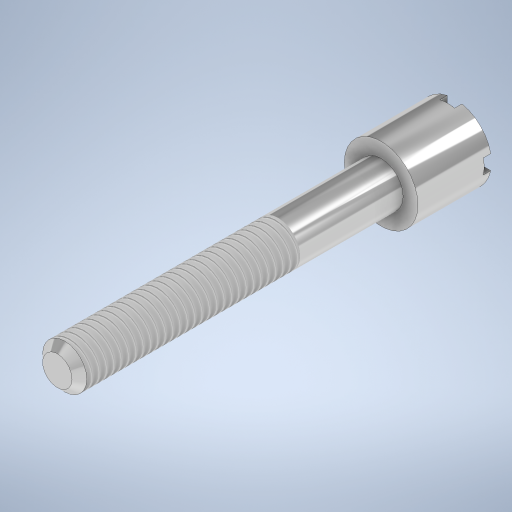
# Autodesk Inventor part: PARAFUSO
Saved by Autodesk Inventor 2023 (Build 270158000, 158)
## iProperties
Created: 2023-10-18
Part Number: PARAFUSO
Material: Genérico
Document SubType Name: Modeling
Designer: vinicius.sena
Density: 1 g/cm^3
Appearance: Padrão
Author: vinicius.sena
Autodesk Inventor part; units mm, degrees
ref_plane "YZ Plane" through (0, 0, 0) normal (1, 0, 0) x (0, 1, 0)
ref_plane "XZ Plane" through (0, 0, 0) normal (0, 1, 0) x (-1, 0, 0)
ref_plane "XY Plane" through (0, 0, 0) normal (0, 0, 1) x (1, 0, 0)
sketch "Esboço1" plane through (0, 0, 0) normal (0, 0, 1) x (1, 0, 0)
  circle A0 centre (0, 0) radius 2.5
  dimension "d0" = 5
  constraints: 1 centre point, 1 coincident
  measures "d0" diameter of A0
extrude "Extrusão1" add sketch "Esboço1" along normal blind 5
sketch "Esboço2" plane through (0, 0, 5) normal (0, 0, 1) x (1, 0, 0)
  circle A0 centre (0, 0) radius 1.5
  dimension "d3" = 3
  constraints: 1 centre point, 1 coincident
  measures "d3" diameter of A0
extrude "Extrusão2" add sketch "Esboço2" along normal blind 22
thread "Rosca1" size "M3x0.5" class "6g" standard "ANSI Metric M Profile" length 15 offset 7
sketch "Esboço3" plane through (0, 0, 0) normal (0, 0, -1) x (-1, 0, 0)
  point P0 (0, 0)
  point P1 (0, 0)
  dimension "d15" = 0
  dimension "d16" = 0
  measures "d15" distance of point (0, 0) point (0, 0)
  measures "d16" distance of point (0, 0) point (0, 0)
hole "Furo1" at (0, 0, 0) direction (0, 0, 1) diameter 2.459 depth 4 tip angle 118 thread size "M3x0.5" class "6H" standard "ANSI Metric M Profile"
sketch "Esboço4" plane through (0, 0, 0) normal (0, 0, -1) x (-1, 0, 0)
  line L0 (-0.5, -3) -> (0.5, -3)
  line L1 (0.5, -3) -> (0.5, 3)
  line L2 (0.5, 3) -> (-0.5, 3)
  line L3 (-0.5, 3) -> (-0.5, -3)
  line L4 (-0.5, -3) -> (0.5, 3) construction
  line L5 (0.5, -3) -> (-0.5, 3) construction
  line L6 (-3, -0.5) -> (3, -0.5)
  line L7 (3, -0.5) -> (3, 0.5)
  line L8 (3, 0.5) -> (-3, 0.5)
  line L9 (-3, 0.5) -> (-3, -0.5)
  line L10 (-3, -0.5) -> (3, 0.5) construction
  line L11 (3, -0.5) -> (-3, 0.5) construction
  point P0 (0, 0)
  point P1 (-0.5, -0.5)
  point P2 (-0.5, 0.5)
  point P3 (0.5, 0.5)
  point P4 (0.5, -0.5)
  dimension "d17" = 1
  dimension "d18" = 6
  dimension "d19" = 6
  dimension "d20" = 1
  constraints: 24 end point, 4 midpoint, 4 parallel, 2 horizontal, 2 perpendicular
  measures "d17" distance of L2.end L1.end
  measures "d18" distance of L1.end L0.end
  measures "d19" distance of L8.end L7.end
  measures "d20" distance of L7.end L6.end
extrude "Extrusão3" cut sketch "Esboço4" against normal blind 0.5 contours L3 L6 L1 L0 | L6 L9 L8 L3 | L1 L8 L7 L6 | L3 L2 L1 L8
chamfer "Chanfro1" distance 1.27 angle 45 3 edges at (0, -1.2295, 0.5) (1.2295, 0, 0.5) (-1.2295, 0, 0.5)
chamfer "Chanfro2" distance 0.5 angle 45 1 edges at (-1.5, 0, 27)
